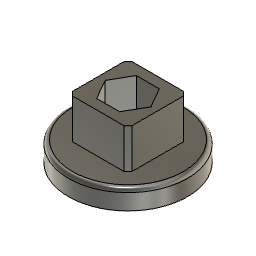
01 (Autodesk Fusion 360 design; units mm, degrees)
Autodesk Fusion 360 part; units mm, degrees
sketch "Sketch1" plane through (0, 0, 0) normal (0, 0, 1) x (1, 0, 0)
  circle A0 centre (0, 0) radius 30
  line L0 (15, 15) -> (-15, 15)
  line L1 (-15, 15) -> (-15, -15)
  line L2 (-15, -15) -> (15, -15)
  line L3 (15, -15) -> (15, 15)
  line L4 (15, 15) -> (-15, -15) construction
  line L5 (-15, 15) -> (15, -15) construction
  dimension "d1" = 60
  dimension "d2" = 30
  dimension "d3" = 30
  constraint coincident A0.centre origin
  constraint horizontal L0
  constraint perpendicular L0 L1
  constraint parallel L0 L2
  constraint parallel L1 L3
  constraint coincident L4 A0.centre
  constraint coincident L5 A0.centre
  measures "d1" diameter of A0
  measures "d2" distance of L1.end L2.end
  measures "d3" distance of L0.end L1.end
extrude "Extrude1" add sketch "Sketch1" along normal blind 10
extrude "Extrude3" add sketch "Sketch1" along normal blind 30 contours L0 L1 L2 L3
sketch "Sketch3" plane through (0, 0, 30) normal (0, 0, 1) x (-1, 0, 0)
  line L0 (5.7735, -10) -> (11.547, 0)
  line L1 (11.547, 0) -> (5.7735, 10)
  line L2 (5.7735, 10) -> (-5.7735, 10)
  line L3 (-5.7735, 10) -> (-11.547, 0)
  line L4 (-11.547, 0) -> (-5.7735, -10)
  line L5 (-5.7735, -10) -> (5.7735, -10)
  dimension "d11" = 20
  dimension "d12" = 23.094
  measures "d11" distance of L2 L5
  measures "d12" distance of L0.end L3.end
extrude "Extrude4" cut sketch "Sketch3" against normal blind 15
sketch "Sketch4" plane through (0, 0, 30) normal (0, 0, 1) x (-1, 0, 0)
  circle A0 centre (0, 0) radius 10
  line L0 (-5.7735, -10) -> (-11.547, 0)
  constraint coincident A0.centre origin
  constraint tangent A0 L0
extrude "Extrude5" cut sketch "Sketch4" against normal blind 55
fillet "Fillet1" radius 2 1 edges at (-27.9698, -10.8485, 10)
chamfer "Chamfer1" distance 2 angle 45 4 edges at (-15, -15, 20) (-15, 15, 20) (15, 15, 20) (15, -15, 20)
sketch "Sketch2" plane through (0, 0, 30) normal (0, 0, 1) x (-1, 0, 0)
  line L0 (0.7735, -12.8868) -> (11.547, -5.7735)
  line L1 (11.547, -5.7735) -> (10.7735, 7.1132)
  line L2 (10.7735, 7.1132) -> (-0.7735, 12.8868)
  line L3 (-0.7735, 12.8868) -> (-11.547, 5.7735)
  line L4 (-11.547, 5.7735) -> (-10.7735, -7.1132)
  line L5 (-10.7735, -7.1132) -> (0.7735, -12.8868)
extrude "Extrude2" [suppressed]
